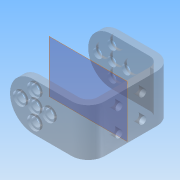
# Autodesk Inventor part: u
Saved by Autodesk Inventor 2015 (Build 190159000, 159)
## iProperties
Created: 2016-01-27
Part Number: u
Material: Plastique PMMA
Document SubType Name: Tôlerie
Designer: Gregwar
Density: 1.188 g/cm^3
Sheet Metal Rule: Par défaut_mm
Appearance: Polycarbonate - Transparent
Author: Gregwar
Autodesk Inventor part; units mm, degrees
ref_plane "YZ Plane" through (0, 0, 0) normal (1, 0, 0) x (0, 1, 0)
ref_plane "XZ Plane" through (0, 0, 0) normal (0, 1, 0) x (-1, 0, 0)
ref_plane "XY Plane" through (0, 0, 0) normal (0, 0, 1) x (1, 0, 0)
sketch "Esquisse6" plane through (20, 29, 10) normal (-1, 0, 0) x (0, 0, 1)
  line L0 (0, -22) -> (-20, -22) construction
  line L1 (-20, -30.3566) -> (-20, -22) construction
  line L2 (0, -30.3566) -> (-20, -30.3566) construction
  line L3 (0, -30.3566) -> (0, -22) construction
  line L4 (-20, 0) -> (0, 0) construction
  line L5 (0, 8.3566) -> (0, 0) construction
  line L6 (-20, 8.3566) -> (0, 8.3566) construction
  line L7 (-20, 8.3566) -> (-20, 0) construction
  line L8 (-20, 8.3566) -> (-20, 0) construction
  line L9 (0, 8.3566) -> (-20, 8.3566) construction
  line L10 (0, 8.3566) -> (0, 0) construction
  line L11 (0, 8.3566) -> (0, 0) construction
  line L12 (-20, -30.3566) -> (-18, -27.6783)
  line L13 (-18, -27.6783) -> (-16, -27.6783)
  line L14 (-16, -27.6783) -> (-16, -24.6783)
  line L15 (-16, -24.6783) -> (-18, -24.6783)
  line L16 (-18, -24.6783) -> (-20, -22)
  line L17 (-20, -30.3566) -> (-20, -22) construction
  line L18 (-20, -26.1783) -> (-16, -26.1783) construction
  line L19 (-20, -22) -> (-20, -30.3566)
  line L20 (-20, -30.3566) -> (0, -30.3566) projected
  line L21 (-10, -22) -> (-10, -30.3566) construction
  line L22 (-20, -22) -> (0, -22) construction
  line L23 (0, -30.3566) -> (0, -22) construction
  line L24 (-20, -30.3566) -> (0, -30.3566) construction
  line L25 (0, -30.3566) -> (-2, -27.6783)
  line L26 (-2, -27.6783) -> (-4, -27.6783)
  line L27 (-4, -27.6783) -> (-4, -24.6783)
  line L28 (-4, -24.6783) -> (-2, -24.6783)
  line L29 (-2, -24.6783) -> (0, -22)
  line L30 (0, -30.3566) -> (0, -22) construction
  line L31 (0, -26.1783) -> (-4, -26.1783) construction
  line L32 (0, -22) -> (0, -30.3566)
  line L33 (0, -30.3566) -> (-20, -30.3566)
  dimension "d31" = 2
  dimension "d32" = 2
  dimension "d33" = 3
  constraints: 48 end point, 10 symmetric about line, 4 midpoint, 3 perpendicular, 2 parallel, 1 vertical
  measures "d31" horizontal distance of L0.end L15.end
  measures "d32" distance of L14.end L15.end
  measures "d33" distance between parallel lines of L13 L15
sketch "Esquisse1" plane through (0, 0, 0) normal (0, 1, 0) x (-1, 0, 0)
  arc A0 (0, -10) -> (0, 10) centre (0, 0) ccw
  line L0 (0, 10) -> (-20, 10)
  line L1 (-20, 10) -> (-20, -10)
  line L2 (-20, -10) -> (0, -10)
  dimension "d0" = 20
  dimension "d1" = 20
  dimension "d2" = 10
  measures "d0" distance between parallel lines of L0 L2
  measures "d1" distance from line of point (0, 0) L1
  measures "d2" radius of A0
extrude "Plaque1" add sketch "Esquisse1" along normal blind 3
sketch "Esquisse2" plane through (0, 0, 0) normal (0, -1, 0) x (1, 0, 0)
  arc A0 (0, 10) -> (0, -10) centre (0, 0) ccw construction
  line L0 (0, 0) -> (-6, 0) construction
  point P0 (0, 6)
  point P1 (0, -6)
  point P2 (6, 0)
  dimension "d6" = 360
  dimension "d8" = 6
  constraints: 3 coincident, 2 end point, 1 horizontal, 5 other
  measures "d8" distance of point (0, 0) point (0, 6)
hole "Perçage1" at (0, 0, 0) at (0, 0, 6) at (-6, 0, 0) at (0, 0, -6) at (6, 0, 0) direction (0, 1, 0) diameter 3.8 end through all counterbore diameter 5.5 counterbore depth 1
ref_plane "Plan de construction1" through (0, 18, 0) normal (0, 1, 0) x (1, 0, 0)
mirror "Symétrie1" about plane through (0, 18, 0) normal (0, 1, 0)
sketch "Esquisse3" plane through (20, 0, 10) normal (1, 0, 0) x (0, 0, -1)
  line L0 (20, 3) -> (0, 3)
  line L1 (0, 0) -> (0, 3)
  line L2 (20, 0) -> (0, 0)
  line L3 (20, 0) -> (20, 3)
  line L4 (20, 33) -> (0, 33)
  line L5 (20, 36) -> (20, 33)
  line L6 (20, 36) -> (0, 36)
  line L7 (0, 36) -> (0, 33)
  line L8 (0, 0) -> (20, 0)
  line L9 (20, 0) -> (20, 36)
  line L10 (20, 36) -> (0, 36)
  line L11 (0, 36) -> (0, 0)
  point P0 (10, 0)
sheet face with bend "Face2" sketch "Esquisse3" thickness 3 toward (1, 0, 0) bend radius 4 relief straight relief width 3 relief depth 1.5 contours L0 L11 L4 L9
bend "Pli1"
sketch "Esquisse4" plane through (23, 0, 10) normal (1, 0, 0) x (0, 0, -1)
  line L0 (20, 7) -> (0, 7) construction
  line L1 (20, 29) -> (20, 7) construction
  line L2 (0, 29) -> (20, 29) construction
  line L3 (0, 7) -> (0, 29) construction
  line L4 (20, 18) -> (0, 18) construction
  circle A0 centre (15, 23) radius 1.5
  line L5 (10, 18) -> (10, 7) construction
  circle A1 centre (15, 13) radius 1.5
  circle A2 centre (5, 23) radius 1.5
  circle A3 centre (5, 13) radius 1.5
  point P0 (10, 0)
  dimension "d22" = 10
  dimension "d23" = 3
  dimension "d25" = 10
  constraints: 4 centre point, 4 end point, 4 midpoint, 3 symmetric about line, 3 other
  measures "d22" distance of A0.centre A1.centre
  measures "d23" diameter of A0
  measures "d25" distance of A2.centre A0.centre
extrude "Couper1" cut sketch "Esquisse4" against normal blind 3
equation "\"d8\" = ollo_spacing"
equation "\"d2\" = 0.5 * d0"
equation "\"d9\" = ollo_hole"
equation "\"d11\" = ollo_ring"
equation "\"d12\" = ollo_depth"
equation "\"d14\" = Epaisseur"
equation "\"d25\" = d22"
equation "\"d26\" = Epaisseur"
equation "\"d17\" = RayonPli"
equation "\"d18\" = LargeurGrugeage"
equation "\"d20\" = RestesMinimum"
equation "\"d19\" = ProfondeurGrugeage"
equation "\"d21\" = RayonPli"
equation "\"LargeurGrugeage\" = Epaisseur"
equation "\"ProfondeurGrugeage\" = 0.5 * Epaisseur"
equation "\"TailleGrugeage\" = 4 * Epaisseur"
equation "\"RestesMinimum\" = 2 * Epaisseur"
equation "\"Rayondetransition\" = RayonPli"
equation "\"TailleRayonJacobi\" = RayonPli"
equation "\"TailleJeu\" = Epaisseur"
equation "\"d3\" = RayonPli"
equation "\"ollo_hole\" = 3.8"
equation "\"ollo_ring\" = 5.5"
equation "\"ollo_depth\" = 1"
equation "\"Epaisseur\" = 3"
equation "\"RayonPli\" = 4"
equation "\"ollo_spacing\" = 6"
